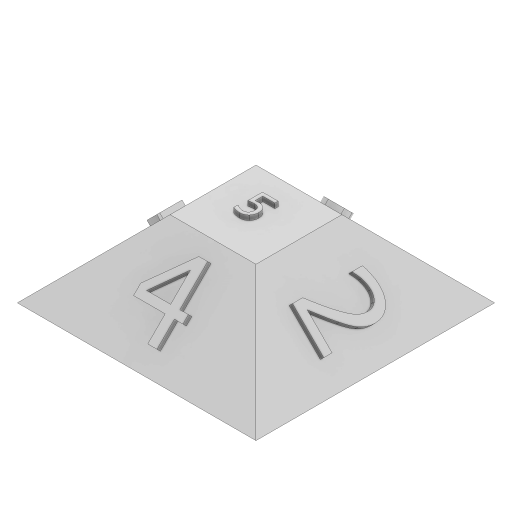
# Autodesk Inventor part: ParcourPyramid
Saved by Autodesk Inventor 2024 (Build 280153000, 153)
## iProperties
Created: 2024-11-28
Part Number: ParcourPyramid
Material: Generisch
Document SubType Name: Modeling
Designer: jonas
Density: 1 g/cm^3
Appearance: Vorgabe
Author: jonas
Autodesk Inventor part; units mm, degrees
ref_plane "YZ Plane" through (0, 0, 0) normal (1, 0, 0) x (0, 1, 0)
sketch "Skizze1" plane through (0, 0, 0) normal (0, 0, 1) x (1, 0, 0)
  line L0 (-25, 0) -> (0, 25)
  line L1 (0, 25) -> (25, 0)
  line L2 (25, 0) -> (-25, 0)
  point P0 (0, 0)
  point P1 (0, 0)
  dimension "d0" = 50
  dimension "d1" = 25
  constraints: 6 end point, 1 coincident, 1 horizontal, 1 midpoint, 1 vertical alignment
  measures "d0" distance of L1.end L0.start
  measures "d1" distance from line of L0.end L2
extrude "Extrusion1" add sketch "Skizze1" along normal blind 50
ref_plane "Arbeitsebene1" through (0, 25, 0) normal (-1, 0, 0) x (0, 0, 1)
sketch "Skizze2" plane through (0, 25, 0) normal (-1, 0, 0) x (0, 0, 1)
  line L0 (0, -25) -> (50, -25) projected
  line L1 (50, -25) -> (25, 0)
  line L2 (0, 0) -> (50, 0) projected
  line L3 (0, -25) -> (25, 0)
  line L4 (0, -25) -> (50, -25)
  line L5 (50, 0) -> (0, 0)
  line L6 (0, 0) -> (0, -25)
  line L7 (0, -25) -> (50, -25)
  line L8 (50, -25) -> (50, 0)
  constraints: 14 end point, 2 horizontal, 2 parallel, 2 perpendicular, 1 midpoint
extrude "Extrusion2" cut sketch "Skizze2" along normal through all both and the other way through all contours L6 L2 L3 | L1 L2 L8
ref_plane "Arbeitsebene2" through (-25, 25, 0) normal (0, -1, 0) x (1, 0, 0)
sketch "Skizze3" plane through (-25, 25, 0) normal (0, -1, 0) x (1, 0, 0)
  line L0 (0, 50) -> (25, 25) projected
  line L1 (0, 50) -> (50, 50)
  line L2 (50, 50) -> (50, 0)
  line L3 (50, 0) -> (0, 0)
  line L4 (0, 0) -> (0, 50)
  point P0 (25, 0)
  constraints: 8 end point, 2 parallel, 1 horizontal, 1 perpendicular
extrude "Extrusion3" cut sketch "Skizze3" along normal blind 9
sketch "Skizze4" plane through (-25, 16, 0) normal (0, 1, 0) x (1, 0, 0)
  line L0 (21.8361, -21.2228) -> (39.593, -21.2228) construction
  line L1 (39.593, -21.2228) -> (39.593, -39.2631) construction
  line L2 (39.593, -39.2631) -> (21.8361, -39.2631) construction
  line L3 (21.8361, -39.2631) -> (21.8361, -21.2228) construction
  spline S0 degree 2 poles (25.9107, -25.3168) (25.9107, -25.7496) (25.6336, -26.4886) (25.3807, -26.7609) knots 0 0 0 1 2 2 2
  spline S1 degree 2 poles (25.3807, -26.7609) (25.1279, -27.0332) (24.3742, -27.3493) (23.9075, -27.3493) knots 0 0 0 1 2 2 2
  spline S2 degree 2 poles (23.9075, -27.3493) (23.4796, -27.3493) (22.6433, -27.1596) (22.337, -27.0089) knots 0 0 0 1 2 2 2
  line L4 (22.337, -27.0089) -> (22.337, -26.158)
  line L5 (22.337, -26.158) -> (22.3953, -26.158)
  spline S3 degree 2 poles (22.3953, -26.158) (22.4877, -26.2261) (22.8329, -26.4011) (23.042, -26.4789) knots 0 0 0 1 2 2 2
  spline S4 degree 2 poles (23.042, -26.4789) (23.2802, -26.5616) (23.6741, -26.654) (23.922, -26.654) knots 0 0 0 1 2 2 2
  spline S5 degree 2 poles (23.922, -26.654) (24.1652, -26.654) (24.6222, -26.4789) (24.7875, -26.2893) knots 0 0 0 1 2 2 2
  spline S6 degree 2 poles (24.7875, -26.2893) (24.9383, -26.1094) (25.0938, -25.6329) (25.0938, -25.312) knots 0 0 0 1 2 2 2
  spline S7 degree 2 poles (25.0938, -25.312) (25.0938, -24.9911) (24.9188, -24.5827) (24.7535, -24.4465) knots 0 0 0 1 2 2 2
  spline S8 degree 2 poles (24.7535, -24.4465) (24.5833, -24.2958) (24.0776, -24.1694) (23.7713, -24.1694) knots 0 0 0 1 2 2 2
  spline S9 degree 2 poles (23.7713, -24.1694) (23.4407, -24.1694) (22.7843, -24.2715) (22.5849, -24.3152) knots 0 0 0 1 2 2 2
  line L6 (22.5849, -24.3152) -> (22.5849, -21.2228)
  line L7 (22.5849, -21.2228) -> (25.8767, -21.2228)
  line L8 (25.8767, -21.2228) -> (25.8767, -21.9279)
  line L9 (25.8767, -21.9279) -> (23.358, -21.9279)
  line L10 (23.358, -21.9279) -> (23.358, -23.5275)
  spline S10 degree 2 poles (23.358, -23.5275) (23.5039, -23.5081) (23.7859, -23.4935) (23.9026, -23.4935) knots 0 0 0 1 2 2 2
  spline S11 degree 2 poles (23.9026, -23.4935) (24.3645, -23.4935) (25.0015, -23.6442) (25.2932, -23.8679) knots 0 0 0 1 2 2 2
  spline S12 degree 2 poles (25.2932, -23.8679) (25.5898, -24.0916) (25.9107, -24.7723) (25.9107, -25.3168) knots 0 0 0 1 2 2 2
  point P0 (25, 0)
  constraints: 2 other
extrude "Extrusion4" add sketch "Skizze4" along normal blind 1
sketch "Skizze5" plane through (-25, 0, 0) normal (-0.7071, 0.7071, 0) x (-0.7071, -0.7071, 0)
  line L0 (-7.7594, 22.2454) -> (-29.861, 22.2454) construction
  line L1 (-29.861, 22.2454) -> (-29.861, 40.4745) construction
  line L2 (-29.861, 40.4745) -> (-7.7594, 40.4745) construction
  line L3 (-7.7594, 40.4745) -> (-7.7594, 22.2454) construction
  line L4 (-11.5957, 28.2648) -> (-8.6686, 28.2648)
  line L5 (-8.6686, 28.2648) -> (-8.6686, 27.6522)
  line L6 (-8.6686, 27.6522) -> (-9.7578, 27.6522)
  line L7 (-9.7578, 27.6522) -> (-9.7578, 23.6311)
  line L8 (-9.7578, 23.6311) -> (-8.6686, 23.6311)
  line L9 (-8.6686, 23.6311) -> (-8.6686, 23.0817)
  spline S0 degree 2 poles (-8.6686, 23.0817) (-9.2861, 23.0817) (-9.8696, 22.7316) (-9.9085, 22.2454) knots 0 0 0 1 2 2 2
  line L10 (-9.9085, 22.2454) -> (-10.5309, 22.2454)
  line L11 (-10.5309, 22.2454) -> (-10.5309, 27.6522)
  line L12 (-10.5309, 27.6522) -> (-11.5957, 27.6522)
  line L13 (-11.5957, 27.6522) -> (-11.5957, 28.2648)
  point P0 (-17.6777, 0)
  constraints: 2 other
extrude "Extrusion5" add sketch "Skizze5" along normal blind 1
sketch "Skizze7" plane through (25, 0, 0) normal (0.7071, 0.7071, 0) x (-0.7071, 0.7071, 0)
  line L0 (15.9722, 17.2103) -> (-5.4407, 17.2103) construction
  line L1 (-5.4407, 17.2103) -> (-5.4407, 35.0228) construction
  line L2 (-5.4407, 35.0228) -> (15.9722, 35.0228) construction
  line L3 (15.9722, 35.0228) -> (15.9722, 17.2103) construction
  line L4 (5.6278, 32.5264) -> (14.8782, 32.5264)
  line L5 (14.8782, 32.5264) -> (14.8782, 30.3991)
  spline S0 degree 2 poles (14.8782, 30.3991) (13.8815, 29.4632) (12.1067, 27.7249) (11.2558, 26.7889) knots 0 0 0 1 2 2 2
  spline S1 degree 2 poles (11.2558, 26.7889) (9.5419, 24.9048) (8.2899, 22.6439) (8.2899, 21.4405) knots 0 0 0 1 2 2 2
  spline S2 degree 2 poles (8.2899, 21.4405) (8.2899, 20.8084) (8.6789, 19.8602) (9.0314, 19.5564) knots 0 0 0 1 2 2 2
  spline S3 degree 2 poles (9.0314, 19.5564) (9.3839, 19.2525) (10.3077, 18.9486) (10.8669, 18.9486) knots 0 0 0 1 2 2 2
  spline S4 degree 2 poles (10.8669, 18.9486) (11.4017, 18.9486) (12.4957, 19.216) (12.9941, 19.4226) knots 0 0 0 1 2 2 2
  spline S5 degree 2 poles (12.9941, 19.4226) (13.4195, 19.5928) (14.2097, 20.079) (14.4528, 20.2492) knots 0 0 0 1 2 2 2
  line L6 (14.4528, 20.2492) -> (14.5622, 20.2492)
  line L7 (14.5622, 20.2492) -> (14.5622, 18.1098)
  spline S6 degree 2 poles (14.5622, 18.1098) (13.9422, 17.806) (11.7178, 17.2103) (10.721, 17.2103) knots 0 0 0 1 2 2 2
  spline S7 degree 2 poles (10.721, 17.2103) (8.6181, 17.2103) (6.2477, 19.4348) (6.2477, 21.3311) knots 0 0 0 1 2 2 2
  spline S8 degree 2 poles (6.2477, 21.3311) (6.2477, 22.2184) (6.661, 23.7014) (7.0257, 24.3335) knots 0 0 0 1 2 2 2
  spline S9 degree 2 poles (7.0257, 24.3335) (7.3904, 24.9899) (8.4479, 26.2784) (9.0314, 26.8983) knots 0 0 0 1 2 2 2
  spline S10 degree 2 poles (9.0314, 26.8983) (9.9795, 27.9316) (12.3012, 30.1439) (12.9941, 30.7881) knots 0 0 0 1 2 2 2
  line L8 (12.9941, 30.7881) -> (5.6278, 30.7881)
  line L9 (5.6278, 30.7881) -> (5.6278, 32.5264)
  point P0 (17.6777, 0)
  constraints: 2 other
extrude "Extrusion6" add sketch "Skizze7" along normal blind 1
sketch "Skizze8" plane through (25, 0, 0) normal (0, 0.7071, -0.7071) x (-1, 0, 0)
  line L0 (28.0899, 7.6104) -> (11.6103, 7.6104) construction
  line L1 (11.6103, 7.6104) -> (11.6103, 24.8911) construction
  line L2 (11.6103, 24.8911) -> (28.0899, 24.8911) construction
  line L3 (28.0899, 24.8911) -> (28.0899, 7.6104) construction
  line L4 (27.7378, 12.0418) -> (27.0015, 11.9457)
  spline S0 degree 2 poles (27.0015, 11.9457) (26.8735, 12.5723) (26.2652, 13.1256) (25.8262, 13.1256) knots 0 0 0 1 2 2 2
  spline S1 degree 2 poles (25.8262, 13.1256) (25.3049, 13.1256) (24.5915, 12.4031) (24.5915, 11.8726) knots 0 0 0 1 2 2 2
  spline S2 degree 2 poles (24.5915, 11.8726) (24.5915, 11.365) (25.2546, 10.7064) (25.7668, 10.7064) knots 0 0 0 1 2 2 2
  spline S3 degree 2 poles (25.7668, 10.7064) (25.9726, 10.7064) (26.2835, 10.7887) knots 0 0 0 1 1 1
  line L5 (26.2835, 10.7887) -> (26.2058, 10.1439)
  spline S4 degree 2 poles (26.2058, 10.1439) (26.128, 10.1531) (26.0869, 10.1531) knots 0 0 0 1 1 1
  spline S5 degree 2 poles (26.0869, 10.1531) (25.6158, 10.1531) (24.8613, 9.6592) (24.8613, 9.1515) knots 0 0 0 1 2 2 2
  spline S6 degree 2 poles (24.8613, 9.1515) (24.8613, 8.7445) (25.4101, 8.214) (25.8445, 8.214) knots 0 0 0 1 2 2 2
  spline S7 degree 2 poles (25.8445, 8.214) (26.2744, 8.214) (26.846, 8.7537) (26.9283, 9.2979) knots 0 0 0 1 2 2 2
  line L6 (26.9283, 9.2979) -> (27.6646, 9.1653)
  spline S8 degree 2 poles (27.6646, 9.1653) (27.5274, 8.4244) (26.5716, 7.6104) (25.8582, 7.6104) knots 0 0 0 1 2 2 2
  spline S9 degree 2 poles (25.8582, 7.6104) (25.3689, 7.6104) (24.5411, 8.0311) (24.1021, 8.7582) (24.1021, 9.1653) knots 0 0 0 1 2 3 3 3
  spline S10 degree 2 poles (24.1021, 9.1653) (24.1021, 9.554) (24.5183, 10.1942) (24.9299, 10.3817) knots 0 0 0 1 2 2 2
  spline S11 degree 2 poles (24.9299, 10.3817) (24.3948, 10.5052) (23.8094, 11.2781) (23.8094, 11.8589) knots 0 0 0 1 2 2 2
  spline S12 degree 2 poles (23.8094, 11.8589) (23.8094, 12.6409) (24.9573, 13.7339) (25.8308, 13.7339) knots 0 0 0 1 2 2 2
  spline S13 degree 2 poles (25.8308, 13.7339) (26.6219, 13.7339) (27.6646, 12.7918) (27.7378, 12.0418) knots 0 0 0 1 2 2 2
  point P0 (25, 0)
  constraints: 2 other
extrude "Extrusion7" add sketch "Skizze8" along normal blind 1
sketch "Skizze9" plane through (-25, 0, 50) normal (0, 0.7071, 0.7071) x (1, 0, 0)
  line L0 (17.9046, 19.3907) -> (35.6431, 19.3907) construction
  line L1 (35.6431, 19.3907) -> (35.6431, -0.0644) construction
  line L2 (35.6431, -0.0644) -> (17.9046, -0.0644) construction
  line L3 (17.9046, -0.0644) -> (17.9046, 19.3907) construction
  line L4 (28.6502, 9.5447) -> (26.8633, 9.5447)
  line L5 (26.8633, 9.5447) -> (26.8633, 4.3907)
  line L6 (26.8633, 4.3907) -> (24.9305, 4.3907)
  line L7 (24.9305, 4.3907) -> (24.9305, 9.5447)
  line L8 (24.9305, 9.5447) -> (18.3057, 9.5447)
  line L9 (18.3057, 9.5447) -> (18.3057, 11.6598)
  line L10 (18.3057, 11.6598) -> (25.0156, 19.3907)
  line L11 (25.0156, 19.3907) -> (26.8633, 19.3907)
  line L12 (26.8633, 19.3907) -> (26.8633, 11.1614)
  line L13 (26.8633, 11.1614) -> (28.6502, 11.1614)
  line L14 (28.6502, 11.1614) -> (28.6502, 9.5447)
  line L15 (24.9305, 11.1614) -> (24.9305, 17.0204)
  line L16 (24.9305, 17.0204) -> (19.886, 11.1614)
  line L17 (19.886, 11.1614) -> (24.9305, 11.1614)
  point P0 (25, 35.3553)
  constraints: 2 other
extrude "Extrusion8" add sketch "Skizze9" along normal blind 1
